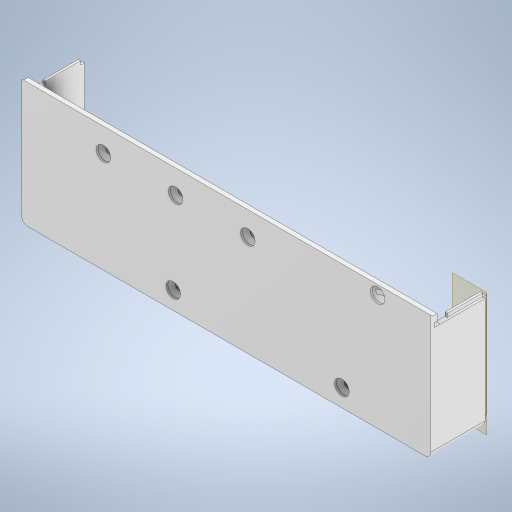
# Autodesk Inventor part: RV_ES_TopLV
Saved by Autodesk Inventor 2023.3 (Build 273359000, 359)
## iProperties
Created: 2023-08-12
Part Number: RV_ES_TopLV
Material: PC/ABS Plastic
Document SubType Name: Modeling
Designer: atrus
Density: 0.357273 g/cm^3
Appearance: Smooth - White
Author: atrus
Autodesk Inventor part; units mm, degrees
ref_plane "YZ Plane" through (0, 0, 0) normal (1, 0, 0) x (0, 1, 0)
ref_plane "XZ Plane" through (0, 0, 0) normal (0, 1, 0) x (-1, 0, 0)
ref_plane "XY Plane" through (0, 0, 0) normal (0, 0, 1) x (1, 0, 0)
ref_plane "Work Plane1" through (0, 65.9695, 5.1) normal (0, 0, 1) x (1, 0, 0)
ref_plane "Work Plane2" through (0, 65.9695, 4.9984) normal (0, 0, 1) x (1, 0, 0)
sketch "Sketch1" plane through (0, 0, 0) normal (0, 0, 1) x (1, 0, 0)
  line L0 (3.175, 0) -> (212.725, 0)
  line L1 (215.9, 59.2341) -> (0, 59.2341)
  line L2 (0, 59.2341) -> (0, 3.175)
  arc A0 (0, 3.175) -> (3.175, 0) centre (3.175, 3.175) ccw
  arc A1 (212.725, 0) -> (215.9, 3.175) centre (212.725, 3.175) ccw
  line L3 (0, 59.2541) -> (183.2664, 59.2541) construction
  line L4 (215.9, 3.175) -> (215.9, 59.2341)
  line L5 (215.9, 3.175) -> (215.9, 128.905) construction
  point P0 (0, 0)
  dimension "d0" = 3.175
  dimension "d3" = 0.02
  constraints: 8 end point, 4 point on circle, 3 tangent, 2 centre point, 2 point on line, 1 collinear, 1 equal radius, 1 horizontal, 1 parallel
  measures "d0" radius of A0
  measures "d3" distance between parallel lines of L1 L3
extrude "Extrusion1" add sketch "Sketch1" along normal up to surface (4.9984 mm away)
sketch "Sketch3" plane through (0, 3.175, 0) normal (-1, 0, 0) x (0, 0, 1)
  line L0 (2.9984, 56.0791) -> (2.9984, 58.0791) construction
  line L1 (2.9984, 58.0791) -> (1.4984, 58.0791) construction
  line L2 (1.4984, 58.0791) -> (1.4984, 61.7945) construction
  line L3 (1.4984, 61.7945) -> (3.9984, 61.7945) construction
  line L4 (3.9984, 61.7945) -> (4.9984, 62.7945) construction
  line L5 (4.9984, 62.6531) -> (4.0398, 61.6945)
  line L6 (4.0398, 61.6945) -> (1.5984, 61.6945)
  line L7 (1.5984, 61.6945) -> (1.5984, 58.1791)
  line L8 (1.5984, 58.1791) -> (3.0984, 58.1791)
  line L9 (3.0984, 58.1791) -> (3.0984, 56.0791)
  line L10 (0, 56.0591) -> (4.9984, 56.0591) projected
  line L11 (4.9984, 56.0591) -> (3.0984, 56.0591)
  line L12 (3.0984, 56.0791) -> (3.0984, 56.0591)
  line L13 (4.9984, 0) -> (4.9984, 56.0591) projected
  line L14 (4.9984, 56.0591) -> (4.9984, 62.6531)
  point P0 (0, -3.175)
  dimension "d4" = 0.1
  dimension "d5" = 0.1
  constraints: 16 end point, 1 parallel, 1 perpendicular, 1 point on line, 3 other
  measures "d4" distance between parallel lines of L4 L5
  measures "d5" distance between parallel lines of L3 L6
extrude "Extrusion2" add sketch "Sketch3" against normal up to surface (215.9 mm away)
ref_plane "Offset Top Of Cable Gland" through (105.029, 1.2065, -5.9716) normal (0, 0, 1) x (1, 0, 0)
ref_plane "Offset from case bottom" through (107.95, 66.04, -23.7516) normal (0, 0, 1) x (1, 0, 0)
sketch "Sketch4" plane through (0, 0, 0) normal (0, 0, -1) x (-1, 0, 0)
  line L0 (-120.915, 0) -> (-120.915, 2.413) construction
  line L1 (-127.265, 2.413) -> (-127.265, 0) construction
  line L2 (-127.265, 2.413) -> (-127.265, 0) construction
  line L3 (-127.265, 0) -> (-136.79, 0) construction
  line L4 (-136.79, 0) -> (-136.79, 2.413) construction
  line L5 (-136.79, 2.413) -> (-127.265, 2.413) construction
  line L6 (-120.915, 0) -> (-120.915, 2.413) construction
  line L7 (-120.915, 2.413) -> (-108.915, 2.413) construction
  line L8 (-108.915, 2.413) -> (-108.915, 0) construction
  line L9 (-108.915, 0) -> (-120.915, 0) construction
  line L10 (-103.835, 0) -> (-103.835, 2.413) construction
  line L11 (-103.835, 2.413) -> (-93.825, 2.413) construction
  line L12 (-93.825, 2.413) -> (-93.825, 0) construction
  line L13 (-93.825, 0) -> (-103.835, 0) construction
  line L14 (-88.745, 0) -> (-88.745, 2.413) construction
  line L15 (-88.745, 2.413) -> (-10.668, 2.413) construction
  line L16 (-10.668, 2.413) -> (-10.668, 0) construction
  line L17 (-10.668, 0) -> (-88.745, 0) construction
  line L18 (-150.66, 2.413) -> (-150.66, 0) construction
  line L19 (-150.66, 0) -> (-199.39, 0) construction
  line L20 (-199.39, 0) -> (-199.39, 1.113) construction
  line L21 (-197.39, 2.413) -> (-150.66, 2.413) construction
  line L22 (-141.87, 2.413) -> (-141.87, 0) construction
  line L23 (-141.87, 0) -> (-145.58, 0) construction
  line L24 (-145.58, 0) -> (-145.58, 2.413) construction
  line L25 (-145.58, 2.413) -> (-141.87, 2.413) construction
  line L26 (-199.49, 0) -> (-199.49, 5.413)
  line L27 (-199.49, 5.413) -> (-10.468, 5.413)
  line L28 (-199.49, 0) -> (-10.468, 0)
  line L29 (-3.175, 0) -> (-212.725, 0) projected
  line L30 (-10.468, 0) -> (-10.468, 5.413)
  line L31 (-197.39, 1.113) -> (-197.39, 2.413) projected
  line L32 (-199.39, 1.113) -> (-197.39, 1.113) projected
  point P0 (0, 0)
  dimension "d8" = 3
  dimension "d23" = 0.1
  dimension "d24" = 0.2
  constraints: 10 end point, 1 perpendicular, 2 other
  measures "d8" distance between parallel lines of L27 L21
  measures "d23" distance between parallel lines of L26 L20
  measures "d24" distance between parallel lines of L30 L16
extrude "CableWall" add sketch "Sketch4" along normal up to surface (5.9716 mm away)
sketch "Sketch5" plane through (199.49, 5.413, -5.9716) normal (0, 0, -1) x (-1, 0, 0)
  line L0 (189.022, 0) -> (0, 0) projected
  line L1 (0, 0) -> (189.122, 0)
  line L2 (189.122, 0) -> (189.122, -2.9)
  line L3 (189.122, -2.9) -> (0, -2.9)
  line L4 (0, -2.9) -> (0, 0)
  line L5 (189.022, -5.413) -> (189.022, 0) construction
  point P0 (199.49, -5.413)
  dimension "d11" = 2.9
  dimension "d39" = 0.1
  constraints: 8 end point, 2 parallel, 1 horizontal, 1 perpendicular
  measures "d11" distance of L1.end L2.end
  measures "d39" distance between parallel lines of L2 L5
extrude "CableInnerLid" add sketch "Sketch5" along normal blind 2
sketch "Sketch6" plane through (3.175, 0, 4.9984) normal (0, -1, 0) x (1, 0, 0)
  arc A0 (85.57, -11.0716) -> (90.65, -11.0716) centre (88.11, -11.0716) ccw construction
  arc A1 (100.66, -11.0716) -> (105.74, -11.0716) centre (103.2, -11.0716) ccw construction
  arc A2 (117.74, -11.0716) -> (124.09, -11.0716) centre (120.915, -11.0716) ccw construction
  arc A3 (133.615, -11.0716) -> (138.695, -11.0716) centre (136.155, -11.0716) ccw construction
  arc A4 (142.405, -11.0716) -> (147.485, -11.0716) centre (144.945, -11.0716) ccw construction
  arc A5 (90.65, -11.0716) -> (85.57, -11.0716) centre (88.11, -11.0716) ccw
  arc A6 (105.74, -11.0716) -> (100.66, -11.0716) centre (103.2, -11.0716) ccw
  arc A7 (124.09, -11.0716) -> (117.74, -11.0716) centre (120.915, -11.0716) ccw
  arc A8 (138.695, -11.0716) -> (133.615, -11.0716) centre (136.155, -11.0716) ccw
  arc A9 (147.485, -11.0716) -> (142.405, -11.0716) centre (144.945, -11.0716) ccw
  line L0 (85.57, -11.0716) -> (85.57, -15.0716)
  line L1 (147.485, -15.0716) -> (147.485, -11.0716)
  line L2 (90.65, -11.0716) -> (90.65, -15.0716)
  line L3 (100.66, -11.0716) -> (100.66, -15.0716)
  line L4 (105.74, -11.0716) -> (105.74, -15.0716)
  line L5 (117.74, -11.0716) -> (117.74, -15.0716)
  line L6 (124.09, -11.0716) -> (124.09, -15.0716)
  line L7 (133.615, -11.0716) -> (133.615, -15.0716)
  line L8 (138.695, -11.0716) -> (138.695, -15.0716)
  line L9 (142.405, -11.0716) -> (142.405, -15.0716)
  line L10 (142.405, -15.0716) -> (147.485, -15.0716)
  line L11 (133.615, -15.0716) -> (138.695, -15.0716)
  line L12 (117.74, -15.0716) -> (124.09, -15.0716)
  line L13 (85.57, -15.0716) -> (90.65, -15.0716)
  line L14 (100.66, -15.0716) -> (105.74, -15.0716)
  line L15 (90.65, -11.0716) -> (88.11, -11.0716) construction
  line L16 (105.74, -11.0716) -> (100.66, -11.0716) construction
  line L17 (124.09, -11.0716) -> (117.74, -11.0716) construction
  line L18 (144.945, -11.0716) -> (142.405, -11.0716) construction
  line L19 (138.695, -11.0716) -> (133.615, -11.0716) construction
  point P0 (-3.175, -4.9984)
  constraints: 50 perpendicular, 40 end point, 14 point on circle, 5 centre point, 5 coincident, 5 concentric, 5 horizontal, 3 tangent, 1 vertical
extrude "CableCutouts" cut sketch "Sketch6" against normal blind 10
sketch "Sketch7" plane through (0, 0, 0) normal (0, 0, -1) x (-1, 0, 0)
  line L0 (-199.39, 2.413) -> (-199.39, 0) construction
  line L1 (-199.49, 0) -> (-212.725, 0) projected
  line L2 (-215.9, 3.175) -> (-215.9, 59.2541) projected
  line L3 (-215.9, 59.2541) -> (-213.487, 59.2541) construction
  line L4 (-213.487, 59.2541) -> (-213.487, 5.588) projected
  arc A0 (-213.487, 5.588) -> (-210.312, 2.413) centre (-210.312, 5.588) ccw projected
  line L5 (-210.312, 2.413) -> (-199.39, 2.413) projected
  line L6 (-199.49, 2.413) -> (-199.49, 0)
  line L7 (-199.49, 0) -> (-212.725, 0) projected
  line L8 (-215.9, 3.175) -> (-215.9, 59.2341) projected
  line L9 (-215.9, 59.1541) -> (-213.487, 59.1541)
  arc A1 (-215.9, 3.175) -> (-212.725, 0) centre (-212.725, 3.175) ccw projected
  line L10 (-212.725, 0) -> (-199.49, 0)
  arc A2 (-5.588, 2.413) -> (-2.413, 5.588) centre (-5.588, 5.588) ccw projected
  line L11 (-2.413, 63.2945) -> (-2.413, 5.588) projected
  arc A3 (-3.175, 0) -> (0, 3.175) centre (-3.175, 3.175) ccw projected
  line L12 (-3.175, 0) -> (-212.725, 0) projected
  line L13 (0, 59.2341) -> (0, 3.175) projected
  line L14 (-10.468, 5.413) -> (-10.468, 0) construction
  line L15 (-1.113, 59.2541) -> (0, 59.2541) construction
  line L16 (-5.588, 2.413) -> (-10.468, 2.413)
  line L17 (-10.468, 2.413) -> (-10.468, 0)
  line L18 (0, 59.1541) -> (-2.413, 59.1541)
  point P0 (-214.6935, 59.1541)
  point P1 (-199.49, 0)
  point P2 (-5.588, 1.113)
  point P3 (-1.113, 5.588)
  dimension "d17" = 0.1
  dimension "d18" = 0.1
  dimension "d41" = 0.1
  dimension "d42" = 0
  constraints: 12 end point, 6 point on line, 3 horizontal, 3 perpendicular, 1 midpoint, 2 other
  measures "d17" vertical distance of L3.end point (-214.693, 59.154)
  measures "d18" distance between parallel lines of L0 L6
  measures "d41" distance between parallel lines of L15 L18
  measures "d42" distance between parallel lines of L14 L17
extrude "SideWallsToBottom" add sketch "Sketch7" along normal up to surface (23.7516 mm away)
sketch "Sketch9" plane through (3.175, 0, 4.9984) normal (0, 0, 1) x (1, 0, 0)
  circle A0 centre (184.785, 60.96) radius 3.45 construction
  circle A1 centre (165.877, 9.398) radius 3.45 construction
  circle A2 centre (76.835, 9.398) radius 3.45 construction
  circle A3 centre (40.005, 53.34) radius 3.45 construction
  circle A4 centre (78.105, 53.34) radius 3.45 construction
  circle A5 centre (116.205, 53.34) radius 3.45 construction
  point P0 (-3.175, 0)
hole "Hole1" at (43.18, 53.34, 4.9984) at (81.28, 53.34, 4.9984) at (80.01, 9.398, 4.9984) at (119.38, 53.34, 4.9984) at (187.96, 60.96, 4.9984) at (169.052, 9.398, 4.9984) direction (0, 0, -1) diameter 3.2766 end through all counterbore diameter 7.62 counterbore depth 3 clearance for "Flat Head Machine Screw (82)" size "#4" standard "Ansi Unified Screw Threads"
chamfer "Chamfer1" distance 2.032 angle 45 8 edges at (187.96, 64.77, 1.9984) (185.9675, 57.7126, 1.9984) (189.9525, 57.7126, 1.9984) (119.38, 57.15, 1.9984) (81.28, 57.15, 1.9984) (43.18, 57.15, 1.9984) (80.01, 13.208, 1.9984) (169.052, 13.208, 1.9984)
sketch "Sketch12" plane through (212.725, 0, -23.7516) normal (0, 0, -1) x (-1, 0, 0)
  line L0 (-0.762, 5.588) -> (-0.762, 59.1541) projected
  arc A0 (-0.762, 5.588) -> (2.413, 2.413) centre (2.413, 5.588) ccw projected
  line L1 (13.235, 2.413) -> (2.413, 2.413) projected
  line L2 (-1.962, 59.1541) -> (-1.962, 5.588)
  arc A1 (-1.962, 5.588) -> (2.413, 1.213) centre (2.413, 5.588) ccw
  line L3 (2.413, 1.213) -> (13.235, 1.213)
  line L4 (13.235, 2.413) -> (13.235, 0) projected
  line L5 (13.235, 1.213) -> (13.235, 2.413)
  line L6 (-0.762, 59.1541) -> (-3.175, 59.1541) projected
  line L7 (-1.962, 59.1541) -> (-0.762, 59.1541)
  arc A2 (207.137, 2.413) -> (210.312, 5.588) centre (207.137, 5.588) ccw projected
  line L8 (207.137, 2.413) -> (202.257, 2.413) projected
  line L9 (210.312, 59.1541) -> (210.312, 5.588) projected
  line L10 (211.512, 59.1541) -> (211.512, 5.588)
  arc A3 (207.137, 1.213) -> (211.512, 5.588) centre (207.137, 5.588) ccw
  line L11 (207.137, 1.213) -> (202.257, 1.213)
  line L12 (210.312, 59.1541) -> (211.512, 59.1541)
  line L13 (210.312, 59.1541) -> (212.725, 59.1541) projected
  line L14 (202.257, 1.213) -> (202.257, 2.413)
  point P0 (212.725, 0)
  dimension "d43" = 1.2
  dimension "d44" = 1.2
  constraints: 16 end point, 4 point on circle, 2 centre point, 1 collinear, 1 horizontal, 1 perpendicular, 1 vertical, 4 other
  measures "d43" distance between parallel lines of L0 L2
  measures "d44" distance between parallel lines of L9 L10
extrude "Extrusion8" add sketch "Sketch12" along normal blind 1.9
sketch "Sketch13" plane through (213.487, 59.1541, 0) normal (0, 1, 0) x (1, 0, 0)
  line L0 (1.2, 23.7516) -> (1.2, 25.6516) projected
  line L1 (1.2, 23.6516) -> (1.2, 5)
  line L2 (0, 0) -> (0, 25.6516) projected
  line L3 (0, 23.6516) -> (1.2, 23.6516)
  line L4 (45.593, 23.7516) -> (-256.667, 23.7516) projected
  line L5 (-212.274, 23.7516) -> (-212.274, 25.6516) construction
  line L6 (-211.074, 0) -> (-213.487, 0)
  line L7 (-211.074, 5) -> (-211.074, 23.6516)
  line L8 (-211.074, 0) -> (-211.074, 25.6516) projected
  line L9 (-212.274, 23.6516) -> (-211.074, 23.6516)
  line L10 (1.2, 5) -> (0, 5)
  line L11 (0, 0) -> (0, 25.6516) projected
  line L12 (0, 5) -> (0, 23.6516)
  line L13 (-211.074, 5) -> (-212.274, 5)
  line L14 (-212.274, 5) -> (-212.274, 23.6516)
  point P0 (0.6, 5)
  dimension "d47" = 0.1
  dimension "d50" = 5
  constraints: 18 end point, 4 collinear, 4 point on line, 3 horizontal, 3 perpendicular, 1 midpoint
  measures "d47" distance between parallel lines of L4 L3
  measures "d50" vertical distance of point (0.6, 5) L2.start
extrude "Extrusion9" add sketch "Sketch13" along normal blind 1.9
body "Solid1"
